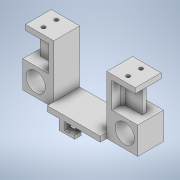
# Autodesk Inventor part: suporte estruzor 1
Saved by Autodesk Inventor 2022 (Build 260153000, 153)
## iProperties
Created: 2022-02-16
Part Number: suporte estruzor 1
Material: Genérico
Document SubType Name: Modeling
Designer: mathe
Density: 1 g/cm^3
Appearance: Padrão
Author: mathe
Autodesk Inventor part; units mm, degrees
ref_plane "YZ Plane" through (0, 0, 0) normal (1, 0, 0) x (0, 1, 0)
ref_plane "XZ Plane" through (0, 0, 0) normal (0, 1, 0) x (-1, 0, 0)
ref_plane "XY Plane" through (0, 0, 0) normal (0, 0, 1) x (1, 0, 0)
sketch "Esboço1" plane through (0, 0, 0) normal (0, 0, 1) x (1, 0, 0)
  line L0 (0, 0) -> (49, 0)
  line L1 (49, 0) -> (49, 41)
  line L2 (0, 41) -> (0, 0)
  line L3 (45, 45) -> (45, 4)
  line L4 (45, 4) -> (4, 4)
  line L5 (4, 4) -> (4, 45)
  line L6 (0, 45) -> (4, 45)
  line L7 (45, 45) -> (49, 45)
  line L8 (45, 45) -> (67, 45)
  line L9 (4, 45) -> (-18, 45)
  line L10 (-18, 45) -> (0, 45)
  line L11 (0, 41) -> (-18, 41)
  line L12 (-18, 41) -> (-18, 45)
  line L13 (67, 45) -> (49, 45)
  line L14 (49, 41) -> (67, 41)
  line L15 (67, 41) -> (67, 45)
  constraints: 32 end point, 5 horizontal, 4 parallel, 2 perpendicular, 1 point on line
extrude "Extrusão1" add sketch "Esboço1" along normal blind 20
sketch "Esboço2" plane through (0, 0, 20) normal (0, 0, 1) x (1, 0, 0)
  line L0 (45, 4) -> (4, 4) projected
  line L1 (0, 0) -> (49, 0) projected
  line L2 (4, 4) -> (45, 4)
  line L3 (45, 4) -> (45, 0)
  line L4 (4, 0) -> (4, 4)
  line L5 (0, 0) -> (49, 0) projected
  line L6 (13.1194, 0) -> (13.1194, -8)
  line L7 (13.1194, -8) -> (23.1194, -8)
  line L8 (23.1194, -8) -> (25.1194, -8)
  line L9 (25.1194, -8) -> (25.1194, -5)
  line L10 (25.1194, -5) -> (21.1194, -5)
  line L11 (21.1194, -5) -> (21.1194, -6)
  line L12 (21.1194, -6) -> (17.1194, -6)
  line L13 (17.1194, -6) -> (17.1194, 0)
  line L14 (45, 0) -> (17.1194, 0)
  line L15 (13.1194, 0) -> (4, 0)
  dimension "d9" = 41
  dimension "d12" = 8
  dimension "d13" = 10
  dimension "d14" = 2
  dimension "d15" = 3
  dimension "d16" = 4
  dimension "d17" = 1
  dimension "d18" = 4
  constraints: 26 end point, 8 perpendicular, 4 point on line, 3 parallel, 1 horizontal
  measures "d9" distance of L3.end L4.start
  measures "d12" distance of L6.start L6.end
  measures "d13" distance of L6.end L7.end
  measures "d14" distance of L7.end L8.end
  measures "d15" distance of L8.end L9.end
  measures "d16" distance of L9.end L10.end
  measures "d17" distance of L10.end L11.end
  measures "d18" distance of L11.end L12.end
extrude "Extrusão2" add sketch "Esboço2" along normal blind 5
sketch "Esboço3" plane through (49, 0, 0) normal (1, 0, 0) x (0, 0, -1)
  line L0 (0, 41) -> (-20, 41) projected
  line L1 (-8.5, 41) -> (-8.5, 21)
  line L2 (-11.5, 41) -> (-11.5, 21)
  line L3 (-11.5, 21) -> (-8.5, 21)
  point P0 (0, 0)
  constraints: 6 end point, 1 horizontal
extrude "Extrusão3" add sketch "Esboço3" along normal blind 15
sketch "Esboço5" plane through (0, 0, 0) normal (-1, 0, 0) x (0, 0, 1)
  line L0 (11.5, 41) -> (11.5, 21) projected
  line L1 (11.5, 41) -> (11.5, 21)
  line L2 (8.5, 21) -> (8.5, 41) projected
  line L3 (11.5, 21) -> (8.5, 21)
  line L4 (8.5, 21) -> (8.5, 41)
  line L5 (8.5, 41) -> (11.5, 41)
  line L6 (0, 41) -> (20, 41) projected
  point P0 (0, 0)
  constraints: 8 end point, 2 collinear, 1 perpendicular, 1 vertical
extrude "Extrusão4" add sketch "Esboço5" along normal blind 15
chamfer "Chanfro1" distance 2 angle 45 8 edges at (49, 31, 11.5) (49, 31, 8.5) (0, 31, 8.5) (0, 31, 11.5) (-7.5, 41, 11.5) (-7.5, 41, 8.5) (56.5, 41, 8.5) (56.5, 41, 11.5)
sketch "Esboço7" plane through (-18, 45, 0) normal (0, 1, 0) x (1, 0, 0)
  line L0 (22, 0) -> (0, 0) projected
  line L1 (22, -20) -> (0, -20) projected
  line L2 (85, -20) -> (63, -20) projected
  line L3 (85, 0) -> (63, 0) projected
  point P0 (18, 0)
  point P1 (9, -15)
  point P2 (9, -5)
  point P3 (74.5, -5)
  point P4 (74.5, -15)
  dimension "d44" = 5
  dimension "d45" = 5
  dimension "d46" = 5
  dimension "d47" = 5
  measures "d44" distance from line of L0 point (9, -5)
  measures "d45" distance from line of L1 point (9, -15)
  measures "d46" distance from line of L2 point (74.5, -15)
  measures "d47" distance from line of L3 point (74.5, -5)
hole "Furo1" at (-9, 45, 15) at (-9, 45, 5) at (56.5, 45, 5) at (56.5, 45, 15) direction (0, -1, 0) diameter 3 end through all
sketch "Esboço8" plane through (0, 0, 20) normal (0, 0, 1) x (1, 0, 0)
  line L0 (0, 0) -> (4, 0) projected
  line L1 (0, 0) -> (-20, 0)
  line L2 (-20, 0) -> (-20, 21)
  line L3 (-20, 21) -> (0, 21)
  line L4 (0, 21) -> (0, 0)
  line L5 (45, 0) -> (49, 0) projected
  line L6 (49, 0) -> (69, 0)
  line L7 (69, 0) -> (69, 21)
  line L8 (69, 21) -> (49, 21)
  line L9 (49, 21) -> (49, 0)
  circle A0 centre (-10, 10.5) radius 7.5
  circle A1 centre (59, 10.5) radius 7.5
  dimension "d38" = 20
  dimension "d39" = 20
  dimension "d40" = 15
  dimension "d41" = 15
  constraints: 16 end point, 4 parallel, 2 centre point, 2 horizontal, 2 perpendicular
  measures "d38" distance of L2.end L3.end
  measures "d39" distance of L8.end L7.end
  measures "d40" diameter of A0
  measures "d41" diameter of A1
extrude "Extrusão6" add sketch "Esboço8" against normal up to surface (20 mm away)
